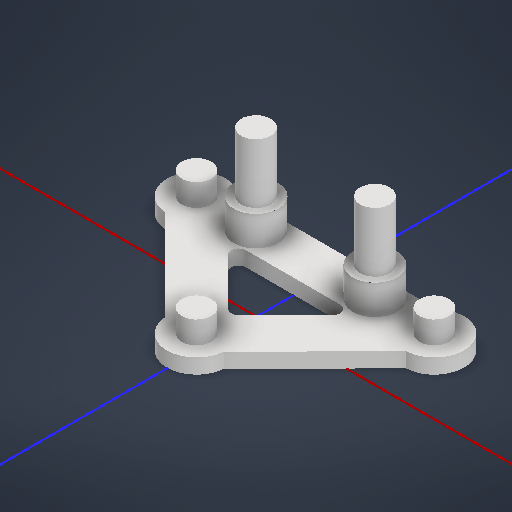
# Autodesk Inventor part: bar
Saved by Autodesk Inventor 2025.4 (Build 294407000, 407)
## iProperties
Created: 2026-09-15
Part Number: bar
Material: Generic
Document SubType Name: Modeling
Designer: User
Density: 1 g/cm^3
Appearance: Default
Author: User
Autodesk Inventor part; units mm, degrees
ref_plane "YZ Plane" through (0, 0, 0) normal (1, 0, 0) x (0, 1, 0)
ref_plane "XZ Plane" through (0, 0, 0) normal (0, 1, 0) x (-1, 0, 0)
ref_plane "XY Plane" through (0, 0, 0) normal (0, 0, 1) x (1, 0, 0)
sketch "Sketch1" plane through (0, 0, 0) normal (0, 1, 0) x (-1, 0, 0)
  line L0 (-8, -4) -> (8, -4)
  line L1 (8, -4) -> (8, 4)
  line L2 (8, 4) -> (-8, 4)
  line L3 (-8, 4) -> (-8, -4)
  line L4 (-8, -4) -> (8, 4) construction
  line L5 (8, -4) -> (-8, 4) construction
  circle A0 centre (8, -4) radius 1
  circle A1 centre (8, -4) radius 2
  circle A2 centre (0, 4) radius 1
  circle A3 centre (-8, -4) radius 1
  circle A4 centre (-8, -4) radius 2
  circle A5 centre (0, 4) radius 2
  line L6 (8, -4) -> (0, 4)
  line L7 (0, 4) -> (-8, -4)
  line L8 (0, -4) -> (0, -5.5)
  line L9 (-6.6771, -5.5) -> (6.6771, -5.5)
  line L10 (4, 0) -> (5.0607, 1.0607)
  line L11 (-4, 0) -> (-5.0607, 1.0607)
  line L12 (0.1252, 5.9961) -> (9.9961, -3.8748)
  line L13 (-8.1282, -2.0445) -> (-1.9931, 4.1658)
  line L14 (-3.5251, -1.6464) -> (-0.3536, 1.5251)
  line L15 (3.5251, -1.6464) -> (0.3536, 1.5251)
  arc A6 (0.3536, 1.5251) -> (-0.3536, 1.5251) centre (0, 1.1716) ccw
  line L16 (3.1716, -2.5) -> (-3.1716, -2.5)
  arc A7 (-3.5251, -1.6464) -> (-3.1716, -2.5) centre (-3.1716, -2) ccw
  arc A8 (3.1716, -2.5) -> (3.5251, -1.6464) centre (3.1716, -2) ccw
  point P0 (0, 0)
  point P1 (0.1252, 5.9961)
  point P2 (-8.0861, -2.0019)
  point P3 (-6.6771, -5.5)
  point P4 (0.1252, 2.0039)
  point P5 (-0.1252, 2.0039)
  point P6 (1.9961, 4.1252)
  point P7 (8.1252, -2.0039)
  dimension "d0" = 16
  dimension "d1" = 8
  dimension "d2" = 2
  dimension "d3" = 4
  dimension "d4" = 2
  dimension "d5" = 2
  dimension "d6" = 4
  dimension "d7" = 4
  dimension "d8" = 1.5
  dimension "d9" = 1.5
  dimension "d10" = 1.5
  dimension "d23" = 90
  dimension "d28" = 90
  dimension "d29" = 0.5
  dimension "d31" = 0.5
  dimension "d32" = 1.5
  dimension "d33" = 1.5
  dimension "d34" = 1.5
  dimension "d35" = 90
  constraints: 34 end point, 11 point on circle, 9 centre point, 9 midpoint, 6 tangent, 4 coincident, 3 horizontal, 2 parallel, 2 point on line, 1 equal radius, 1 perpendicular, 1 vertical
  measures "d0" distance of L2.end L1.end
  measures "d1" distance of L1.end L0.end
  measures "d2" diameter of A0
  measures "d3" diameter of A1
  measures "d4" diameter of A2
  measures "d5" diameter of A3
  measures "d6" diameter of A4
  measures "d7" diameter of A5
  measures "d8" distance of L8.start L8.end
  measures "d9" distance of L10.start L10.end
  measures "d10" distance of L11.start L11.end
  measures "d23" angle of L11 L7
  measures "d28" angle of L10 L6
  measures "d29" radius of A6
  measures "d31" radius of A7
  measures "d32" distance between parallel lines of L7 L14
  measures "d33" distance between parallel lines of L6 L15
  measures "d34" distance between parallel lines of L0 L16
  measures "d35" angle of L10 L12
extrude "Extrusion1" add sketch "Sketch1" along normal blind 1 contours A3 L7 A4 L0 | L0 A4 L3 A3 | L3 A4 L7 A3 | A4 L7 A5 L6 A1 L0 | L0 L8 L9 A4 | A4 L13 L3 | L3 L13 L11 L7 A4 | L0 A1 L9 L8 | L11 L13 L2 A5 L7 | A1 L6 A0 L0 | L0 A0 L1 A1 L12 | L7 A2 L6 A5 | A5 L2 A2 L7 | L6 L10 L12 L1 A1 | A1 L1 A0 L6 | L13 A5 L2 | A5 L12 L2 A2 | L6 A2 L2 A5 | A5 L2 L12 L10 L6 | L1 L12 A1 | A5 L12 L2 | A1 L12 | A5 L12
sketch "Sketch2" plane through (0, 1, 0) normal (0, 1, 0) x (1, 0, 0)
  line L0 (-8.1252, 2.0039) -> (-1.9961, -4.1252) projected
  arc A0 (-1.9961, -4.1252) -> (1.9931, -4.1658) centre (0, -4) ccw projected
  line L1 (1.9931, -4.1658) -> (8.0861, 2.0019) projected
  arc A1 (8.0861, 2.0019) -> (6.6771, 5.5) centre (8, 4) ccw projected
  line L2 (6.6771, 5.5) -> (-6.6771, 5.5) projected
  arc A2 (-6.6771, 5.5) -> (-8.1252, 2.0039) centre (-8, 4) ccw projected
  circle A3 centre (-8, 4) radius 1 projected
  circle A4 centre (0, -4) radius 1 projected
  circle A5 centre (8, 4) radius 1 projected
  point P0 (0, 0)
extrude "Extrusion2" add sketch "Sketch2" along normal blind 1.5 and the other way blind 1 contours A3 | A5
sketch "Sketch4" plane through (0, 1, 0) normal (0, 1, 0) x (1, 0, 0)
  line L0 (-8.1252, 2.0039) -> (-1.9961, -4.1252) projected
  arc A0 (-1.9961, -4.1252) -> (1.9931, -4.1658) centre (0, -4) ccw projected
  line L1 (1.9931, -4.1658) -> (8.0861, 2.0019) projected
  arc A1 (8.0861, 2.0019) -> (6.6771, 5.5) centre (8, 4) ccw projected
  line L2 (6.6771, 5.5) -> (-6.6771, 5.5) projected
  arc A2 (-6.6771, 5.5) -> (-8.1252, 2.0039) centre (-8, 4) ccw projected
  circle A3 centre (-8, 4) radius 1 projected
  circle A4 centre (8, 4) radius 1 projected
  circle A5 centre (0, -4) radius 1 projected
  line L3 (-3.1716, 2.5) -> (3.1716, 2.5) projected
  arc A6 (3.5251, 1.6464) -> (3.1716, 2.5) centre (3.1716, 2) ccw projected
  line L4 (3.5251, 1.6464) -> (0.3536, -1.5251) projected
  arc A7 (-0.3536, -1.5251) -> (0.3536, -1.5251) centre (0, -1.1716) ccw projected
  line L5 (-0.3536, -1.5251) -> (-3.5251, 1.6464) projected
  arc A8 (-3.1716, 2.5) -> (-3.5251, 1.6464) centre (-3.1716, 2) ccw projected
  point P0 (0, 0)
extrude "Extrusion4" add sketch "Sketch4" along normal blind 1.5 and the other way blind 1 contours A5
sketch "Sketch5" plane through (0, 1, 0) normal (0, 1, 0) x (1, 0, 0)
  line L0 (-8.1252, 2.0039) -> (-1.9961, -4.1252) projected
  arc A0 (-1.9961, -4.1252) -> (1.9931, -4.1658) centre (0, -4) ccw projected
  line L1 (1.9931, -4.1658) -> (8.0861, 2.0019) projected
  arc A1 (8.0861, 2.0019) -> (6.6771, 5.5) centre (8, 4) ccw projected
  line L2 (6.6771, 5.5) -> (-6.6771, 5.5) projected
  arc A2 (-6.6771, 5.5) -> (-8.1252, 2.0039) centre (-8, 4) ccw projected
  circle A3 centre (-8, 4) radius 1 projected
  circle A4 centre (8, 4) radius 1 projected
  circle A5 centre (0, -4) radius 1 projected
  line L3 (-3.1716, 2.5) -> (3.1716, 2.5) projected
  arc A6 (3.5251, 1.6464) -> (3.1716, 2.5) centre (3.1716, 2) ccw projected
  line L4 (3.5251, 1.6464) -> (0.3536, -1.5251) projected
  arc A7 (-0.3536, -1.5251) -> (0.3536, -1.5251) centre (0, -1.1716) ccw projected
  line L5 (-0.3536, -1.5251) -> (-3.5251, 1.6464) projected
  arc A8 (-3.1716, 2.5) -> (-3.5251, 1.6464) centre (-3.1716, 2) ccw projected
  circle A9 centre (-4, 4) radius 1.5
  circle A10 centre (4, 4) radius 1.5
  point P0 (0, 0)
  dimension "d40" = 3
  dimension "d42" = 4
  dimension "d43" = 4
  dimension "d44" = 1.5
  dimension "d45" = 1.5
  constraints: 2 centre point, 1 equal radius
  measures "d40" diameter of A9
  measures "d42" distance of A3.centre A9.centre
  measures "d43" distance of A4.centre A10.centre
  measures "d44" distance from line of L2 A9.centre
  measures "d45" distance from line of L2 A10.centre
extrude "Extrusion5" add sketch "Sketch5" along normal blind 2 contours A10 | A9
sketch "Sketch6" plane through (-4, 3, -4) normal (0, 1, 0) x (1, 0, 0)
  circle A0 centre (0, 0) radius 1.5 projected
  circle A1 centre (8, 0) radius 1.5 projected
  circle A2 centre (0, 0) radius 1
  circle A3 centre (8, 0) radius 1
  point P0 (4, -4)
  dimension "d48" = 2
  dimension "d49" = 2
  constraints: 2 centre point, 2 coincident
  measures "d48" diameter of A2
  measures "d49" diameter of A3
extrude "Extrusion6" add sketch "Sketch6" along normal blind 4 contours A2 | A3
equation "\"d2\" = d4"
equation "\"d3\" = d7"
equation "\"d5\" = d4"
equation "\"d6\" = d7"
equation "\"d45\" = d44"
equation "\"d49\" = d48"
body "Solid1"
